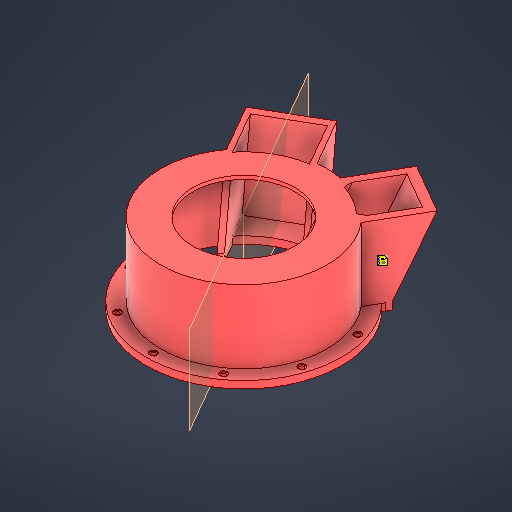
# Autodesk Inventor part: Thermal Housing
Saved by Autodesk Inventor 2026.2 (Build 302298000, 298)
## iProperties
Created: 2025-12-15
Part Number: Thermal Housing
Material: ABS Plastic
Document SubType Name: Modeling
Designer: mayhe
Density: 1.06 g/cm^3
Appearance: Smooth - White
Author: mayhe
Autodesk Inventor part; units mm, degrees
ref_plane "XZ Plane" through (0, 0, 0) normal (0, 1, 0) x (-1, 0, 0)
ref_plane "XY Plane" through (0, 0, 0) normal (0, 0, 1) x (1, 0, 0)
sketch "Sketch1" plane through (0, 0, 0) normal (0, 1, 0) x (-1, 0, 0)
  circle A0 centre (0, 0) radius 135
  circle A1 centre (0, 0) radius 110.125
  circle A2 centre (0, 0) radius 115
  line L0 (-32.8125, -134.8329) -> (-100.3625, -95.8329)
  line L1 (-100.3625, -95.8329) -> (-77.5375, -56.2989)
  line L2 (-77.5375, -56.2989) -> (-9.9875, -95.2989)
  line L3 (-9.9875, -95.2989) -> (-31.5625, -132.6679)
  line L4 (-32.8125, -134.8329) -> (-31.5625, -132.6679)
  line L5 (100.25, -95.6381) -> (100.25, -95.6381)
  line L6 (132.95, 39) -> (132.95, 39)
  line L7 (-43.7625, -75.7989) -> (-66.5875, -115.3329)
  line L8 (-88.95, -76.0659) -> (-20.775, -113.9834)
  line L9 (4.0985, -98.6989) -> (83.4265, -52.8989)
  line L10 (83.4265, -52.8989) -> (106.2515, -92.4329)
  line L11 (106.2515, -92.4329) -> (26.9235, -138.2329)
  line L12 (26.9235, -138.2329) -> (4.0985, -98.6989)
  line L13 (4.0985, -98.6989) -> (106.2515, -92.4329) construction
  line L14 (83.4265, -52.8989) -> (26.9235, -138.2329) construction
  point P0 (0, -135)
  point P1 (-30.847, -131.4285)
  point P2 (-98.397, -92.4285)
  point P3 (39, -130.675)
  point P4 (-17.719, -108.6902)
  point P5 (-20.3175, -113.191)
  point P6 (-87.8675, -74.191)
  point P7 (-85.269, -69.6902)
  point P8 (-85.7464, -104.2715)
  point P9 (-47.4286, -126.3943)
  point P10 (116.9134, -67.5)
  point P11 (-54.8625, -95.0246)
  point P12 (0, -110.35)
  point P13 (13.0792, -114.2538)
  point P14 (92.4071, -68.4538)
  point P15 (85.7464, -104.2715)
  point P16 (103.1607, -87.0796)
  point P17 (23.8328, -132.8796)
  point P18 (47.4286, -126.3943)
  point P19 (-44.9878, -100.5167)
  point P20 (-61.6641, -91.2417)
  point P21 (89.7386, -63.8318)
  point P22 (10.4107, -109.6318)
  dimension "d0" = 270
  dimension "d1" = 220.25
  dimension "d10" = 4.875
  dimension "d17" = 78
  dimension "d107" = 78
  dimension "d292" = 91.6
  dimension "d293" = 45.65
  dimension "d295" = 133.175
  constraints: 30 end point, 5 midpoint, 4 parallel, 3 coincident, 2 centre point, 2 perpendicular, 1 vertical alignment, 3 other
  measures "d1" diameter of A1
  measures "d10" radial gap between concentric circles of A1 A2
  measures "d17" distance of L1.end L2.end
  measures "d107" distance of L0.start L0.end
  measures "d292" distance of L10.end L11.end
  measures "d293" distance of L9.end L10.end
  measures "d295" distance from line of L11 point (0, 0)
extrude "Cylinder Base" add sketch "Sketch1" along normal blind 10 contours A0 L10 A2 L1 | L1 L8 A2 L7 L0 A0 | A0 L0 L1 | L10 L11 A0 | A0 L11 L12 A2 L10 | L1 A2 L8 | L10 A1 L1 A2 | A2 L12 A1 L10 | L0 L7 A2 L8 L3 A0 | A0 L3 L4 L0 | L1 A1 L8 A2 | L8 A1 L7 A2 | L11 L12 A0 | L12 A0 L3 A2 | A2 L3 A1 L12 | L7 A1 L8 A2 | L3 L8 A2 | A2 L8 A1 L3
extrude "Cylinder Walls" add sketch "Sketch1" along normal blind 110.5 contours L10 A1 L1 A2 | A2 L3 A1 L12
sketch "Sketch4" plane through (0, 110.5, 0) normal (0, 1, 0) x (1, 0, 0)
  circle A0 centre (0, 0) radius 110.125
  circle A1 centre (0, 0) radius 70.375
  dimension "d27" = 140.75
  constraints: 2 centre point, 2 coincident
  measures "d27" diameter of A1
extrude "Cylinder Top" add sketch "Sketch4" against normal blind 5
sketch "Thermal" plane through (0, 110.5, 0) normal (0, 1, 0) x (1, 0, 0)
  line L0 (87.8675, 74.191) -> (126.275, 140.7147)
  line L1 (126.275, 140.7147) -> (58.725, 179.7147)
  line L2 (58.725, 179.7147) -> (20.3175, 113.191)
  line L3 (61.223, 164.0413) -> (111.4524, 135.0413)
  line L4 (111.4524, 135.0413) -> (83.9524, 87.4099)
  line L5 (83.9524, 87.4099) -> (25.0627, 121.4099)
  line L6 (33.723, 116.4099) -> (61.223, 164.0413)
  line L7 (61.223, 164.0413) -> (83.9524, 87.4099) construction
  line L8 (111.4524, 135.0413) -> (33.723, 116.4099) construction
  arc A0 (33.723, 116.4099) -> (83.9524, 87.4099) centre (64.1433, 111.0995) ccw
  line L9 (85.269, 69.6902) -> (87.8675, 74.191)
  line L10 (87.8675, 74.191) -> (85.269, 69.6902)
  line L11 (20.3175, 113.191) -> (17.719, 108.6902)
  line L12 (17.719, 108.6902) -> (20.3175, 113.191)
  line L13 (18.5627, 110.1516) -> (13.5627, 101.4913)
  line L14 (13.5627, 101.4913) -> (81.1127, 62.4913)
  line L15 (81.1127, 62.4913) -> (85.269, 69.6902)
  line L16 (83.9524, 87.4099) -> (92.6127, 82.4099)
  line L17 (59.521, 170.3933) -> (117.8045, 136.7433)
  line L18 (117.8045, 136.7433) -> (87.5823, 84.397)
  arc A1 (29.2988, 118.047) -> (87.5823, 84.397) centre (64.1433, 111.0995) ccw
  line L19 (29.2988, 118.047) -> (59.521, 170.3933)
  arc A2 (85.269, 69.6902) -> (17.719, 108.6902) centre (0, 0) ccw projected
  line L20 (87.8675, 74.191) -> (85.269, 69.6902) projected
  line L21 (17.719, 108.6902) -> (20.3175, 113.191) projected
  point P0 (56.7125, 98.2289)
  point P1 (72.5877, 125.7256)
  point P2 (17.9287, 109.0535)
  point P3 (28.7645, 107.8215)
  point P4 (78.2337, 77.5048)
  point P5 (37.3618, 87.7509)
  point P6 (57.3136, 76.2317)
  point P7 (29.696, 118.7349)
  point P8 (87.9795, 85.0849)
  point P9 (78.9939, 78.8215)
  point P10 (33.9183, 104.7715)
  point P11 (73.7756, 81.7598)
  point P12 (100.3625, 95.8329)
  point P13 (32.8125, 134.8329)
  dimension "d33" = 78
  dimension "d36" = 55
  dimension "d115" = 10
  dimension "d132" = 78
  dimension "d133" = 10
  dimension "d134" = 23
  dimension "d135" = 4.65
  dimension "d150" = 10
  dimension "d284" = 185
  constraints: 40 end point, 6 point on circle, 3 point on line, 2 centre point, 2 midpoint
  measures "d33" distance between parallel lines of L2 L0
  measures "d36" distance of L3.end L4.end
  measures "d115" distance between parallel lines of L4 L0
  measures "d132" distance of L14.end L13.end
  measures "d133" distance of L13.end L13.start
  measures "d134" distance between parallel lines of L14 L5
  measures "d135" distance between parallel lines of L6 L19
  measures "d150" distance between parallel lines of L6 L2
  measures "d284" distance from line of point (0, 0) L1
ref_plane "Work Plane6" through (0, 0, 0) normal (0.8660254, 0, 0.5) x (0, 1, 0)
sketch "Sweep (Thermal)" plane through (0, 0, 0) normal (0.8660254, 0, 0.5) x (0, 1, 0)
  line L0 (10, -133.175) -> (110.5, -178.433)
  line L1 (0, -129.244) -> (0, -103.1607) projected
  line L2 (10, -133.175) -> (0, -133.175)
  point P0 (0, 0)
  point P1 (0, -30.847)
  dimension "d283" = 65.757
  constraints: 4 end point
  measures "d283" angle of L1 L0
sweep "Thermal Sweep" add profiles "Thermal" path "Sweep (Thermal)" keep normal constant yes path curves L0 L2 contours L9 A2 A1 L18 L16 L0 | L16 L18 L17 L19 L5 L2 L1 L0 | L18 A1 A2 A0 L16 | L16 L4 L3 L6 L5 L19 L17 L18 | L5 L19 A1 A2 L11 L2 | A0 A2 A1 L19 L5
ref_plane "Work Plane5" through (0, 0, 0) normal (0.8660254, 0, -0.5) x (0, 1, 0)
sketch "Optical" plane through (0, 110.5, 0) normal (0, 1, 0) x (1, 0, 0)
  line L0 (-89.7386, 63.8318) -> (-129.664, 132.9846)
  line L1 (-129.664, 132.9846) -> (-50.336, 178.7846)
  line L2 (-10.4107, 109.6318) -> (-13.0792, 114.2538) projected
  line L3 (-10.4107, 109.6318) -> (-50.336, 178.7846)
  line L4 (-118.775, 127.7243) -> (-85.269, 69.6902)
  line L5 (-17.719, 108.6902) -> (-51.225, 166.7243)
  line L6 (-51.225, 166.7243) -> (-118.775, 127.7243)
  arc A0 (-85.269, 69.6902) -> (-89.7386, 63.8318) centre (0, 0) ccw
  arc A1 (-10.4107, 109.6318) -> (-17.719, 108.6902) centre (0, 0) ccw
  point P0 (-83.4, 144.453)
  dimension "d299" = 91.6
  dimension "d301" = 6.8
  dimension "d302" = 78
  dimension "d306" = 180
  dimension "d307" = 170
  constraints: 12 end point, 4 point on circle, 2 centre point, 2 parallel, 2 perpendicular, 1 coincident, 1 collinear
  measures "d299" distance of L0.end L1.end
  measures "d301" distance between parallel lines of L0 L4
  measures "d302" distance of L5.end L4.start
  measures "d306" distance from line of L1 point (0, 0)
  measures "d307" distance from line of point (0, 0) L6
sketch "Sweep (Optical)" plane through (0, 0, 0) normal (0.8660254, 0, -0.5) x (0, 1, 0)
  line L0 (0, -133.175) -> (10, -133.175)
  line L1 (10, -133.175) -> (110.5, -163.6673)
  point P0 (0, 0)
  constraints: 4 end point
sweep "Optical Sweep" add profiles "Optical" path "Sweep (Optical)" keep normal constant yes path curves L1 L0
sketch "Sketch20" plane through (0, 10, 0) normal (0, 1, 0) x (1, 0, 0)
  circle A0 centre (0, 0) radius 125
  circle A1 centre (0, -125) radius 2.5
  circle A2 centre (73.4732, -101.1271) radius 2.5
  circle A3 centre (118.8821, -38.6271) radius 2.5
  circle A4 centre (118.8821, 38.6271) radius 2.5
  circle A5 centre (73.4732, 101.1271) radius 2.5
  circle A6 centre (0, 125) radius 2.5
  circle A7 centre (-73.4732, 101.1271) radius 2.5
  circle A8 centre (-118.8821, 38.6271) radius 2.5
  circle A9 centre (-118.8821, -38.6271) radius 2.5
  circle A10 centre (-73.4732, -101.1271) radius 2.5
  dimension "d136" = 250
  dimension "d137" = 5
  dimension "d140" = 360
  constraints: 10 centre point, 1 coincident, 1 vertical alignment, 23 other
  measures "d137" diameter of A1
hole "Hole3" at (118.8821, 10, -38.6271) at (118.8821, 10, 38.6271) at (73.4732, 10, 101.1271) at (0, 10, 125) at (-73.4732, 10, 101.1271) at (-118.8821, 10, 38.6271) at (-118.8821, 10, -38.6271) at (0, 10, -125) direction (0, -1, 0) diameter 5.9 depth 10 tip angle 118 counterbore diameter 10.2 counterbore depth 1.2
sketch "Sketch31" plane through (0, 0, 0) normal (1, 0, 0) x (0, 1, 0)
  line L0 (0, -129.2475) -> (0, -131.4285) projected
  line L1 (0, -114) -> (2.5, -114)
  line L2 (2.5, -114) -> (2.5, -117)
  line L3 (2.5, -117) -> (0, -117)
  line L4 (0, -117) -> (0, -114)
  line L5 (-0.5, 0) -> (3, 0) projected
  point P0 (0, 0)
  point P1 (0, -115.5)
  point P2 (0, -117)
  point P3 (0, -129.244)
  point P4 (0, 16.2648)
  point P5 (0, -126.3943)
  point P6 (0, -92.4285)
  point P7 (0, -92.4285)
  point P8 (0, -131.4285)
  point P9 (0, -132.8796)
  point P10 (0, -87.0796)
  dimension "d211" = 2.5
  dimension "d212" = 3
  dimension "d260" = 114
  constraints: 8 end point, 2 parallel, 1 horizontal, 1 midpoint, 1 perpendicular, 2 other
  measures "d211" distance of L2.end L3.end
  measures "d212" distance of L1.end L2.end
  measures "d260" distance from line of point (0, 0) L1
revolve "Seal Groove" cut sketch "Sketch31" angle 360 about axis through (0, -10, 0) along (0, 1, 0)
sketch "Sketch43" plane through (0, 0, 0) normal (0, -1, 0) x (1, 0, 0)
  line L0 (-32.8125, -134.8329) -> (-100.3625, -95.8329) projected
  line L1 (-32.8125, -134.8329) -> (-35.9789, -140.3172) projected
  line L2 (-35.9789, -140.3172) -> (-103.5289, -101.3172) projected
  line L3 (-103.5289, -101.3172) -> (-100.3625, -95.8329) projected
  point P0 (0, 0)
extrude "Extrusion30" add sketch "Sketch43" against normal up to surface (10 mm away)
body "Solid1"
